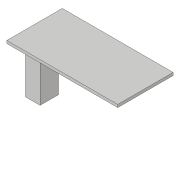
# Autodesk Inventor part: Part6
Saved by Autodesk Inventor 2019 (Build 230136000, 136)
## iProperties
Created: 2019-11-12
Part Number: Part6
Material: Generic
Document SubType Name: Sheet Metal
Designer: Mahesh
Density: 1 g/cm^3
Sheet Metal Rule: Default
Appearance: Default
Author: Mahesh
Autodesk Inventor part; units mm, degrees
ref_plane "YZ Plane" through (0, 0, 0) normal (1, 0, 0) x (0, 1, 0)
ref_plane "XZ Plane" through (0, 0, 0) normal (0, 1, 0) x (-1, 0, 0)
ref_plane "XY Plane" through (0, 0, 0) normal (0, 0, 1) x (1, 0, 0)
sketch "Sketch1" plane through (0, 0, 0) normal (0, 1, 0) x (-1, 0, 0)
  line L0 (1000, 0) -> (1000, -0.5649)
  line L1 (1000, -0.5649) -> (0, -0.5649)
  line L2 (0, -0.5649) -> (0, 0)
  line L3 (0, -0.5649) -> (-2000, -0.5649)
  line L4 (-2000, -0.5649) -> (-2000, 999.4351)
  line L5 (-2000, 999.4351) -> (0, 999.4351)
  line L6 (0, 999.4351) -> (0, -0.5649)
  dimension "d1" = 2000
  dimension "d2" = 1000
  constraints: 14 end point, 2 parallel, 1 horizontal, 1 perpendicular
  measures "d1" distance of L4.end L5.end
  measures "d2" distance of L3.end L4.end
extrude "Extrusion1" add sketch "Sketch1" along normal blind 50
sketch "Sketch2" plane through (0, 0, 0) normal (0, -1, 0) x (1, 0, 0)
  point P0 (0, 0)
sketch "Sketch3" plane through (0, 0, 0) normal (0, -1, 0) x (1, 0, 0)
  line L0 (98.4679, 994.5253) -> (98.4679, 664.5253)
  line L1 (98.4679, 330.5706) -> (98.4679, 0)
  line L2 (0, -0.5649) -> (0, 999.4351) projected
  line L3 (0, 664.5253) -> (264.4565, 664.5253)
  line L4 (264.4565, 664.5253) -> (264.4565, 330.5706)
  line L5 (264.4565, 330.5706) -> (0, 330.5706)
  line L6 (0, 330.5706) -> (0, 664.5253)
  point P0 (0, 0)
  dimension "d5" = 330
  constraints: 12 end point, 2 parallel, 2 vertical, 1 horizontal, 1 perpendicular, 1 point on line
  measures "d5" distance of L0.start L0.end
extrude "Extrusion2" add sketch "Sketch3" along normal blind 1000
sketch "Sketch4" plane through (0, -1000, 0) normal (0, -1, 0) x (1, 0, 0)
  line L0 (0, 664.5253) -> (264.4565, 664.5253) projected
  line L1 (132.2283, 664.5253) -> (132.2283, 497.5253)
  circle A0 centre (132.2283, 497.5253) radius 100
  point P0 (0, 0)
  dimension "d8" = 167
  dimension "d9" = 200
  constraints: 2 end point, 1 centre point, 1 coincident, 1 midpoint, 1 vertical
  measures "d8" distance of L1.start L1.end
  measures "d9" diameter of A0
extrude "Extrusion3" cut sketch "Sketch4" against normal blind 100
sketch "Sketch5" plane through (0, 0, 0) normal (0, -1, 0) x (1, 0, 0)
  point P0 (0, 0)
equation "\"BendRadius\" = Thickness"
equation "\"BendReliefWidth\" = Thickness"
equation "\"BendReliefDepth\" = 0.5 * Thickness"
equation "\"CornerReliefSize\" = 4 * Thickness"
equation "\"MinimumRemnant\" = 2 * Thickness"
equation "\"TransitionRadius\" = BendRadius"
equation "\"JacobiRadiusSize\" = BendRadius"
equation "\"GapSize\" = Thickness"
equation "\"Thickness\" = 3.048"
body "Solid1"
